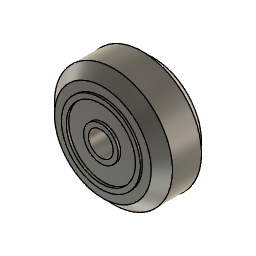
V slot wheel D23.9 v2 (Autodesk Fusion 360 design; units mm, degrees)
Autodesk Fusion 360 part; units mm, degrees
sketch "Sketch1" plane through (0, 0, 0) normal (0, 1, 0) x (1, 0, 0)
  circle A0 centre (0, 0) radius 11.95
  circle A1 centre (0, 0) radius 9.8
  circle A2 centre (0, 0) radius 8
  circle A3 centre (0, 0) radius 2.5
  circle A4 centre (0, 0) radius 7
  circle A5 centre (0, 0) radius 3.5
  dimension "d1" = 23.9
  dimension "d2" = 19.6
  dimension "d3" = 16
  dimension "d4" = 5
  dimension "d13" = 14
  dimension "d14" = 7
  constraint coincident A0.centre A1.centre
  constraint concentric A0 A1
  constraint concentric A1 A2
  constraint concentric A1 A4
  constraint concentric A1 A5
  measures "d1" diameter of A0
  measures "d2" diameter of A1
  measures "d3" diameter of A2
  measures "d4" diameter of A3
  measures "d13" diameter of A4
  measures "d14" diameter of A5
extrude "Extrude3" add sketch "Sketch1" along normal mid plane 10.2 contours A0 | A1 makes body 1
chamfer "Chamfer1" distance 2.15 distance2 2.15 2 edges at (-11.1413, -5.1, -4.3213) (-11.1413, 5.1, 4.3213) measured on face at (10.5888, -5.1, 0.5937) measured on face at (10.5888, 5.1, 0.5937) on bodies 1
extrude "Extrude4" add sketch "Sketch1" along normal mid plane 11 separate body contours A2 | A5 makes body 2 at (7.9901, 3.6667, 0.3988) makes body 3 at (3.4956, 3.6667, 0.1745)
extrude "Extrude5" add sketch "Sketch1" along normal mid plane 10 contours A4 bodies 2 3
named bodies: "Body1", "Body2"
